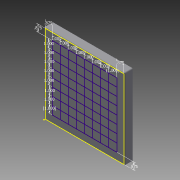
# Autodesk Inventor part: chess-board
Saved by Autodesk Inventor 2014 (Build 180170000, 170)
## iProperties
Created: 2014-12-29
Part Number: chess-board
Material: Generic
Document SubType Name: Modeling
Designer: TechShop Member
Density: 1 g/cm^3
Appearance: Default
Author: TechShop Member
Autodesk Inventor part; units mm, degrees
ref_plane "YZ Plane" through (0, 0, 0) normal (1, 0, 0) x (0, 1, 0)
ref_plane "XZ Plane" through (0, 0, 0) normal (0, 1, 0) x (-1, 0, 0)
ref_plane "XY Plane" through (0, 0, 0) normal (0, 0, 1) x (1, 0, 0)
sketch "Sketch1" plane through (0, 0, 0) normal (0, 0, 1) x (1, 0, 0)
  line L0 (0, 0) -> (254, 0)
  line L1 (254, 0) -> (254, 254)
  line L2 (254, 254) -> (0, 254)
  line L3 (0, 254) -> (0, 0)
  dimension "d0" = 254
  dimension "d1" = 254
  constraints: 8 end point, 2 parallel, 1 horizontal, 1 perpendicular
  measures "d0" distance of L1.end L2.end
  measures "d1" distance of L0.end L1.end
extrude "Extrusion1" add sketch "Sketch1" along normal blind 25.4
fillet "Fillet1" radius 3.175 1 edges at (127, 254, 25.4)
fillet "Fillet2" radius 3.175 3 edges at (0, 253.0701, 24.4701) (0, 254, 11.1125) (0, 125.4125, 25.4)
fillet "Fillet3" radius 3.175 3 edges at (254, 253.0701, 24.4701) (254, 254, 11.1125) (254, 125.4125, 25.4)
fillet "Fillet4" radius 3.175 5 edges at (253.0701, 0, 24.4701) (254, 0, 11.1125) (0.9299, 0, 24.4701) (0, 0, 11.1125) (127, 0, 25.4)
sketch "Sketch2" plane through (0, 0, 25.4) normal (0, 0, 1) x (1, 0, 0)
  line L0 (250.825, 3.175) -> (3.175, 3.175) projected
  line L1 (250.825, 250.825) -> (250.825, 3.175) projected
  line L2 (3.175, 250.825) -> (250.825, 250.825) projected
  line L3 (3.175, 3.175) -> (3.175, 250.825) projected
  line L4 (25.4, 25.4) -> (25.4, 228.6)
  line L5 (25.4, 228.6) -> (228.6, 228.6)
  line L6 (228.6, 228.6) -> (228.6, 25.4)
  line L7 (228.6, 25.4) -> (25.4, 25.4)
  line L8 (50.8, 228.6) -> (50.8, 25.4)
  line L9 (203.2, 228.6) -> (203.2, 25.4)
  line L10 (177.8, 228.6) -> (177.8, 25.4)
  line L11 (76.2, 228.6) -> (76.2, 25.4)
  line L12 (101.6, 228.6) -> (101.6, 25.4)
  line L13 (152.4, 228.6) -> (152.4, 25.4)
  line L14 (127, 228.6) -> (127, 25.4)
  line L15 (25.4, 50.8) -> (228.6, 50.8)
  line L16 (25.4, 76.2) -> (228.6, 76.2)
  line L17 (25.4, 203.2) -> (228.6, 203.2)
  line L18 (25.4, 177.8) -> (228.6, 177.8)
  line L19 (25.4, 152.4) -> (228.6, 152.4)
  line L20 (25.4, 127) -> (228.6, 127)
  line L21 (25.4, 101.6) -> (228.6, 101.6)
  point P0 (0, 0)
  dimension "d8" = 22.225
  dimension "d9" = 22.225
  dimension "d10" = 22.225
  dimension "d11" = 22.225
  dimension "d12" = 25.4
  dimension "d13" = 25.4
  dimension "d14" = 25.4
  dimension "d15" = 25.4
  dimension "d16" = 25.4
  dimension "d17" = 25.4
  dimension "d18" = 25.4
  dimension "d19" = 25.4
  dimension "d20" = 25.4
  dimension "d21" = 25.4
  dimension "d22" = 25.4
  dimension "d23" = 25.4
  dimension "d24" = 25.4
  dimension "d25" = 25.4
  dimension "d26" = 25.4
  dimension "d27" = 25.4
  constraints: 28 end point, 10 vertical, 7 horizontal, 40 other
  measures "d13" distance between parallel lines of L8 L11
  measures "d14" distance between parallel lines of L12 L11
  measures "d15" distance between parallel lines of L14 L12
  measures "d16" distance between parallel lines of L13 L14
  measures "d17" distance between parallel lines of L10 L13
  measures "d18" distance between parallel lines of L9 L10
  measures "d21" distance between parallel lines of L18 L17
  measures "d22" distance between parallel lines of L19 L18
  measures "d23" distance between parallel lines of L20 L19
  measures "d24" distance between parallel lines of L21 L20
  measures "d25" distance between parallel lines of L16 L21
  measures "d26" distance between parallel lines of L15 L16
body "Solid1"
